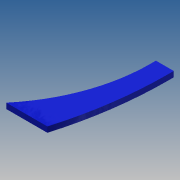
# Autodesk Inventor part: UA-072-PlatteLinks
Saved by Autodesk Inventor 2015 (Build 190159000, 159)
## iProperties
Created: 2014-09-09
Part Number: UA-072-PlatteLinks
Material: Allgemein
Document SubType Name: Modeling
Designer: Semenov
Density: 1 g/cm^3
Appearance: Blau - Wandfarbe - glänzend
Author: Semenov
Autodesk Inventor part; units mm, degrees
ref_plane "YZ Plane" through (0, 0, 0) normal (1, 0, 0) x (0, 1, 0)
ref_plane "XZ Plane" through (0, 0, 0) normal (0, 1, 0) x (-1, 0, 0)
ref_plane "XY Plane" through (0, 0, 0) normal (0, 0, 1) x (1, 0, 0)
sketch "Skizze3" plane through (0, 0, 0) normal (0, 0, 1) x (1, 0, 0)
  line L0 (-500, 500) -> (500, 500)
  line L1 (500, 500) -> (500, -500)
  line L2 (500, -500) -> (-500, -500)
  line L3 (-500, -500) -> (-500, 500)
  line L4 (-500, -400) -> (500, -400)
  line L5 (-275, 500) -> (275, 500)
  line L6 (275, 500) -> (275, 320)
  line L7 (275, 320) -> (-275, 320)
  line L8 (-275, 320) -> (-275, 500)
  arc A0 (-275, 320) -> (-400, -400) centre (1736.1, -400) ccw
  arc A1 (400, -400) -> (275, 320) centre (-1736.1, -400) ccw
  line L9 (-160, 320) -> (160, 320)
  line L10 (160, 320) -> (160, 360)
  line L11 (160, 360) -> (-160, 360)
  line L12 (-160, 360) -> (-160, 320)
  line L13 (-440, -450) -> (-140, -450)
  line L14 (90, -450) -> (440, -450)
  line L15 (-30, 360) -> (-30, 320)
  arc A2 (-440, -450) -> (-160, 320) centre (-1358.75, 320) ccw
  arc A3 (-140, -450) -> (-30, 320) centre (-2780, 320) ccw
  arc A4 (-30, 320) -> (90, -450) centre (2500.4167, 320) ccw
  arc A5 (160, 320) -> (440, -450) centre (1358.75, 320) ccw
  line L16 (-160, 360) -> (-440, -450) construction
  line L17 (-160, 360) -> (-146.1239, 400.1416) construction
  line L18 (-30, 360) -> (-146.1239, 400.1416) construction
  line L19 (-30, 360) -> (121.8543, 307.5071) construction
  line L20 (-440, -450) -> (-172.0218, -542.6344) construction
  line L21 (-140, -450) -> (-172.0218, -542.6344) construction
  line L22 (-140, -450) -> (121.8543, 307.5071) construction
  line L23 (-172.9217, 310.595) -> (139.7195, 418.6685) construction
  line L24 (139.7195, 418.6685) -> (440, -450) construction
  line L25 (440, -450) -> (127.3587, -558.0735) construction
  line L26 (127.3587, -558.0735) -> (-172.9217, 310.595) construction
  point P0 (0, 0)
  point P1 (-500, 0)
  point P2 (0, 500)
  point P3 (0, 320)
  point P4 (0, 360)
  dimension "d4" = 1000
  dimension "d5" = 1000
  dimension "d6" = 100
  dimension "d7" = 550
  dimension "d8" = 180
  dimension "d9" = 100
  dimension "d10" = 100
  dimension "d11" = 320
  dimension "d12" = 300
  dimension "d13" = 350
  dimension "d14" = 230
  dimension "d15" = 60
  dimension "d16" = -60
  dimension "d17" = 130
  dimension "d18" = 190
  dimension "d19" = 50
  dimension "d21" = 283.5374
  dimension "d22" = 40
  dimension "d23" = 140
  dimension "d24" = 899.502
  dimension "d25" = 919.1046
  dimension "d26" = 330.7937
  constraints: 54 end point, 12 point on circle, 11 perpendicular, 11 point on line, 8 parallel, 6 centre point, 4 midpoint, 4 tangent, 3 collinear, 3 horizontal, 3 vertical alignment, 2 horizontal alignment, 2 line through centre
  measures "d4" distance of L0.start L0.end
  measures "d5" distance of L2.end L0.start
  measures "d6" distance between parallel lines of L2 L4
  measures "d7" distance of L6.end L7.end
  measures "d8" distance of L5.end L6.end
  measures "d9" distance from line of A0.end L3
  measures "d10" distance from line of A1.start L1
  measures "d11" distance of L10.end L11.end
  measures "d12" distance of L13.start L13.end
  measures "d13" distance of L14.end L14.start
  measures "d14" distance of L14.start L13.end
  measures "d15" distance from line of L13.start L3
  measures "d16" distance from line of L14.end L1
  measures "d17" distance between parallel lines of L15 L12
  measures "d18" distance between parallel lines of L15 L10
  measures "d19" distance between parallel lines of L14 L2
  measures "d21" distance between parallel lines of L21 L16
  measures "d22" distance between parallel lines of L9 L11
  measures "d23" distance between parallel lines of L11 L0
  measures "d24" distance between parallel lines of L20 L18
  measures "d25" distance between parallel lines of L25 L23
  measures "d26" distance between parallel lines of L24 L26
extrude "Extrusion6" add sketch "Skizze3" along normal blind 40 contours A2 A0 L4 | L4 A3 L13 A2 | L12 L11 L15 L7 | L7 A3 L4 A0 A2
equation "\"d9\" = d6"
equation "\"d10\" = d6"
